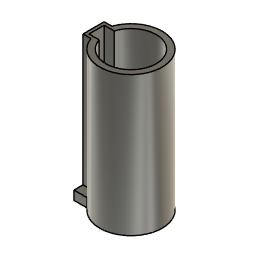
v1 (Autodesk Fusion 360 design; units mm, degrees)
Autodesk Fusion 360 part; units mm, degrees
sketch "Skizze1" plane through (0, 0, 0) normal (0, 0, 1) x (1, 0, 0)
  line L0 (-8.1311, 2.477) -> (-11.4995, 2.477)
  line L1 (-11.4995, 2.477) -> (-11.4995, -2.6586)
  line L2 (-11.4995, -2.6586) -> (-8.0735, -2.6586)
  line L3 (-5.4995, 2.477) -> (-11.4995, -2.6586) construction
  line L4 (-11.4995, 2.477) -> (-5.4995, -2.6586) construction
  line L5 (-9.9076, 3.477) -> (-12.5, 3.477)
  line L6 (-12.5, 3.477) -> (-12.5, -3.5)
  line L7 (-9.842, -3.6586) -> (-12.5, -3.6586)
  line L8 (-12.5, -3.6586) -> (-9.2883, -3.6586)
  line L9 (-12.5, -3.5) -> (-12.5, -3.6586)
  arc A0 (-9.842, -3.6586) -> (-9.9076, 3.477) centre (0, 0) ccw
  arc A1 (-8.0735, -2.6586) -> (-8.1311, 2.477) centre (0, 0) ccw
  dimension "d1" = 17
  dimension "d2" = 21
  dimension "d3" = 6
  constraint coincident A0.centre A1.centre
  constraint concentric A0 A1
  constraint horizontal L0
  constraint perpendicular L0 L1
  constraint parallel L0 L2
  constraint perpendicular L5 L6
  constraint parallel L7 L8
  constraint perpendicular L8 L9
  measures "d1" diameter of A1
  measures "d2" diameter of A0
  measures "d3" distance of L1.end L4.end
extrude "Extrusion1" add sketch "Skizze1" along normal blind 41
sketch "Skizze2" plane through (0, 0, 0) normal (0, 0, -1) x (1, 0, 0)
  arc A0 (-8.1311, -2.477) -> (-8.0735, 2.6586) centre (0, 0) ccw
  line L0 (-8.1311, -2.477) -> (-11.4995, -2.477)
  line L1 (-11.4995, -2.477) -> (-11.4995, 2.6586)
  line L2 (-11.4995, 2.6586) -> (-8.0735, 2.6586)
  arc A1 (-9.9076, -3.477) -> (-9.842, 3.6586) centre (0, 0) ccw
  line L3 (-9.842, 3.6586) -> (-12.5, 3.6586)
  line L4 (-12.5, 3.6586) -> (-12.5, -3.477)
  line L5 (-12.5, -3.477) -> (-9.9076, -3.477)
  circle A2 centre (0, 0) radius 14.6163
  constraint coincident A0.centre A1.centre
extrude "Extrusion2" add sketch "Skizze2" along normal blind 6 contours A0 L0 L1 L2 | A1 L3 L4 L5
sketch "Skizze3" plane through (0, 0, -6) normal (0, 0, -1) x (1, 0, 0)
  line L0 (-12.5, -3.477) -> (-9.9076, -3.477)
  arc A0 (-9.9076, -3.477) -> (-9.842, 3.6586) centre (0, 0) ccw
  line L1 (-9.842, 3.6586) -> (-12.5, 3.6586)
  line L2 (-12.5, 3.6586) -> (-12.5, -3.477)
  line L3 (-7, 3) -> (7, 3)
  line L4 (7, 3) -> (7, -3)
  line L5 (7, -3) -> (-7, -3)
  line L6 (-7, -3) -> (-7, 3)
  line L7 (-7, 3) -> (7, -3) construction
  line L8 (7, 3) -> (-7, -3) construction
  line L9 (-2, 3) -> (2, 3)
  line L10 (2, 3) -> (2, -3)
  line L11 (2, -3) -> (-2, -3)
  line L12 (-2, -3) -> (-2, 3)
  line L13 (-2, 3) -> (2, -3) construction
  line L14 (2, 3) -> (-2, -3) construction
  constraint horizontal L3
  constraint perpendicular L3 L4
  constraint parallel L3 L5
  constraint parallel L4 L6
  constraint coincident L7 A0.centre
  constraint coincident L8 A0.centre
  constraint coincident A0.centre origin
  constraint horizontal L9
  constraint perpendicular L9 L10
  constraint parallel L9 L11
  constraint parallel L10 L12
  constraint coincident L13 A0.centre
  constraint coincident L14 A0.centre
  constraint coincident L3 L9.start
extrude "Extrusion3" cut sketch "Skizze3" against normal blind 5 contours L3 L5 L6 L12 | L3 L4 L5 L10
sketch "Skizze4" plane through (-2, 0, 0) normal (-1, 0, 0) x (0, -1, 0)
  line L0 (-3, -6) -> (3, -6)
  line L1 (3, -6) -> (3, -1)
  line L2 (3, -1) -> (-3, -1)
  line L3 (-3, -1) -> (-3, -6)
  line L4 (3, -1) -> (-3, -1)
  line L5 (-3, -1) -> (-3, -4)
  line L6 (-3, -4) -> (3, -4)
  line L7 (3, -4) -> (3, -1)
  dimension "d12" = 6
  constraint horizontal L4
  constraint vertical L5
  constraint horizontal L6
  constraint vertical L7
  constraint coincident L1.end L2.start
  measures "d12" distance of L1.end L2.end
extrude "Extrusion4" cut sketch "Skizze4" against normal blind 6 contours L1 L2 L3 L4 L5 L6 L7
fillet "Abrundung1" radius 5.5 2 edges at (-7, 0, -1) (7, 0, -1)
sketch "Skizze5" plane through (0, 0, -6) normal (0, 0, -1) x (1, 0, 0)
  line L0 (-2, 3) -> (-2, -3)
  line L1 (-2, -3) -> (-7, -3)
  line L2 (-7, -3) -> (-7, 3)
  line L3 (-7, 3) -> (-2, 3)
  line L4 (2, -3) -> (2, 3)
  line L5 (2, 3) -> (7, 3)
  line L6 (7, 3) -> (7, -3)
  line L7 (7, -3) -> (2, -3)
  line L8 (-12.5, -3.477) -> (-9.9076, -3.477)
  arc A0 (-9.9076, -3.477) -> (-9.842, 3.6586) centre (0, 0) ccw
  line L9 (-9.842, 3.6586) -> (-12.5, 3.6586)
  line L10 (-12.5, 3.6586) -> (-12.5, -3.477)
  line L11 (-7.973, -6.5355) -> (-17.027, -6.5355)
  line L12 (-17.027, -6.5355) -> (-17.027, 6.7171)
  line L13 (-17.027, 6.7171) -> (-7.973, 6.7171)
  line L14 (-7.973, 6.7171) -> (-7.973, -6.5355)
  line L15 (-7.973, -6.5355) -> (-17.027, 6.7171) construction
  line L16 (-17.027, -6.5355) -> (-7.973, 6.7171) construction
  line L17 (-12.5, -3.477) -> (-12.5, -6.5355)
  line L18 (-12.5, 3.6586) -> (-12.5, 6.8537)
  point P0 (-12.5, 0.0908)
  constraint horizontal L11
  constraint perpendicular L11 L12
  constraint parallel L11 L13
  constraint parallel L12 L14
  constraint coincident L15 P0
  constraint coincident L16 P0
  constraint midpoint L10 P0
  constraint coincident L8.start L10.end
  constraint midpoint L11 L17.end
  constraint coincident L9.end L10.start
  constraint perpendicular L13 L18
extrude "Extrusion5" add sketch "Skizze5" against normal blind 3 contours L8 A0 L11 L17 | A0 L9 L13 L18
sketch "Skizze6" plane through (0, 0, 0) normal (0, 0, 1) x (-1, 0, 0)
  line L0 (8.1311, -2.477) -> (11.4995, -2.477)
  line L1 (11.4995, -2.477) -> (11.4995, 2.6586)
  line L2 (11.4995, 2.6586) -> (8.0735, 2.6586)
  arc A0 (8.0735, 2.6586) -> (8.1311, -2.477) centre (0, 0) ccw
  circle A1 centre (0, 0) radius 6.5199
  line L3 (0, 0) -> (8.1311, -2.477)
  line L4 (0, 0) -> (8.0735, 2.6586)
  constraint coincident A0.centre A1.centre
  constraint coincident L0.start A0.end
  constraint coincident L2.end A0.start
extrude "Extrusion6" add sketch "Skizze6" along normal blind 1.6 contours A0 A1 L3 L4
